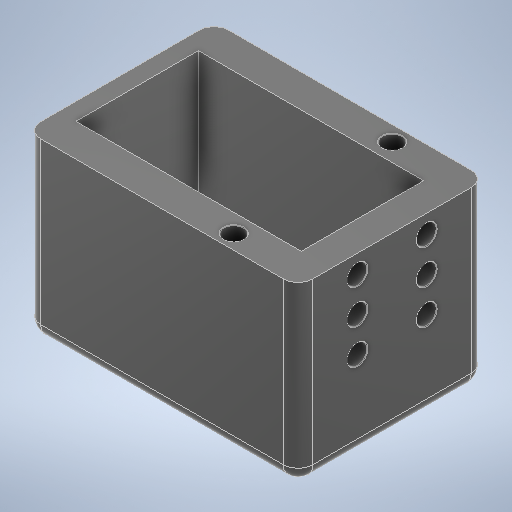
# Autodesk Inventor part: basketback
Saved by Autodesk Inventor 2025.3 (Build 293356000, 356)
## iProperties
Created: 2026-04-05
Part Number: basketback
Material: PCTG 20%
Document SubType Name: Modeling
Designer: ksawe
Density: 1.541 g/cm^3
Appearance: Smooth - Black
Author: ksawe
Autodesk Inventor part; units mm, degrees
ref_plane "YZ Plane" through (0, 0, 0) normal (1, 0, 0) x (0, 1, 0)
ref_plane "XZ Plane" through (0, 0, 0) normal (0, 1, 0) x (-1, 0, 0)
ref_plane "XY Plane" through (0, 0, 0) normal (0, 0, 1) x (1, 0, 0)
sketch "Sketch1" plane through (0, 0, 0) normal (0, 1, 0) x (-1, 0, 0)
  line L0 (22.75, -10.36) -> (7.75, -10.36)
  line L1 (7.75, -10.36) -> (-0.1031, 0)
  circle A0 centre (4.34, -10.36) radius 1
  line L2 (22.75, 10.36) -> (7.75, 10.36)
  circle A1 centre (12.64, 0) radius 9.6 construction
  line L3 (22.75, 12.36) -> (22.75, -12.36)
  circle A2 centre (4.34, 10.36) radius 1
  line L4 (7.75, 10.36) -> (-0.1031, 0)
  line L5 (26.25, 19) -> (26.25, -19)
  line L6 (22.75, -12.36) -> (-22.75, -12.36)
  line L7 (22.75, 0) -> (-22.75, 0) construction
  line L8 (26.25, -19) -> (-28.75, -19)
  line L9 (26.25, -19) -> (-28.75, 19) construction
  line L10 (-28.75, -19) -> (26.25, 19) construction
  line L11 (-22.75, 12.36) -> (22.75, 12.36)
  line L12 (-28.75, 19) -> (26.25, 19)
  line L13 (-28.75, -19) -> (-28.75, 19)
  circle A3 centre (-16.36, 10.25) radius 1
  line L14 (-22.75, -12.36) -> (-22.75, 12.36)
  circle A4 centre (-16.36, -10.25) radius 1
  point P0 (0, 0)
  point P1 (-1.25, 0)
  point P2 (0, 0)
  point P3 (22.75, -10.36)
  dimension "d0" = 55
  dimension "d1" = 38
  dimension "d2" = 45.5
  dimension "d3" = 24.72
  dimension "d4" = 2
  dimension "d6" = 18.41
  dimension "d7" = 20.5
  dimension "d8" = 19.2
  dimension "d9" = 10.11
  dimension "d10" = 13
  dimension "d11" = 15
  dimension "d12" = 3.5
  dimension "d13" = 2
  dimension "d68" = 3.41
  dimension "d69" = 20.7
  constraints: 30 end point, 5 centre point, 5 midpoint, 4 parallel, 4 symmetric about line, 3 horizontal, 3 point on line, 2 coincident, 2 perpendicular, 1 equal radius, 1 horizontal alignment, 3 other
  measures "d0" distance of L9.end L5.start
  measures "d1" distance of L8.end L9.end
  measures "d2" distance of L11.start L3.start
  measures "d3" distance of L6.end L11.start
  measures "d4" diameter of A2
  measures "d6" distance from line of L3 A2.centre
  measures "d7" distance of A3.centre A4.centre
  measures "d8" diameter of A1
  measures "d9" distance from line of L3 A1.centre
  measures "d10" distance of L2.end L1.end
  measures "d11" distance of L2.start L2.end
  measures "d12" distance between parallel lines of L5 L3
  measures "d13" distance between parallel lines of L11 L2
  measures "d68" distance of L2.end A2.centre
  measures "d69" horizontal distance of A3.centre A2.centre
extrude "Extrusion1" add sketch "Sketch1" along normal mid plane 1 contours L3 L6 L14 L11 L2 L4 L1 L0 | L5 L8 L13 L12
extrude "Extrusion2" add sketch "Sketch1" along normal blind 35 contours L5 L8 L13 L12
fillet "Fillet1" radius 3 8 edges at (1.25, -0.5, -19) (28.75, -0.5, 0) (1.25, -0.5, 19) (-26.25, -0.5, 0) (28.75, 17.25, -19) (28.75, 17.25, 19) (-26.25, 17.25, 19) (-26.25, 17.25, -19)
sketch "Sketch6" plane through (28.75, 2.5, 16) normal (1, 0, 0) x (0, 0, -1)
  circle A0 centre (23, 14.75) radius 1.5
  line L0 (0, 32.5) -> (32, 32.5) projected
  line L1 (16, 32.5) -> (16, 0)
  line L2 (32, 0) -> (0, 0) projected
  line L3 (16, 39.5) -> (16, 7)
  circle A1 centre (23, 21.75) radius 1.5
  line L4 (16, 46.5) -> (16, 14)
  circle A2 centre (23, 28.75) radius 1.5
  line L5 (2, 32.5) -> (2, 0)
  circle A3 centre (9, 14.75) radius 1.5
  line L6 (2, 39.5) -> (2, 7)
  circle A4 centre (9, 21.75) radius 1.5
  line L7 (2, 46.5) -> (2, 14)
  circle A5 centre (9, 28.75) radius 1.5
  point P0 (16, -2.5)
  dimension "d50" = 3
  dimension "d54" = 7
  dimension "d57" = 14
  dimension "d70" = 3.75
  constraints: 12 end point, 6 centre point, 2 midpoint, 1 collinear, 1 horizontal, 1 vertical, 25 other
  measures "d50" diameter of A0
  measures "d54" distance of L1.start L3.start
  measures "d57" distance of L1.start L5.start
  measures "d70" distance from line of L0 A5.centre
hole "Hole2" at (28.75, 31.25, 7) at (28.75, 31.25, -7) at (28.75, 24.25, -7) at (28.75, 24.25, 7) at (28.75, 17.25, 7) at (28.75, 17.25, -7) direction (-1, 0, 0) diameter 4 depth 5 countersink diameter 4.2 countersink angle 90
sketch "Sketch7" plane through (0, 35, 0) normal (0, 1, 0) x (1, 0, 0)
  line L0 (-26.25, 16) -> (-26.25, -16) projected
  line L1 (-26.25, 0) -> (28.75, 0)
  line L2 (28.75, -16) -> (28.75, 16) projected
  line L3 (-23.25, -16) -> (25.75, -16) projected
  circle A0 centre (12.75, -16) radius 1.5
  circle A1 centre (12.75, 16) radius 1.5
  point P0 (0, 0)
  dimension "d71" = 3
  dimension "d72" = 16
  constraints: 2 centre point, 2 end point, 2 midpoint, 1 point on line, 1 symmetric about line, 1 other
  measures "d71" diameter of A0
  measures "d72" distance from line of L2 A0.centre
hole "Hole3" at (12.75, 35, 16) at (12.75, 35, -16) direction (0, -1, 0) diameter 4 depth 7 countersink diameter 4.2 countersink angle 90
body "Solid1"
